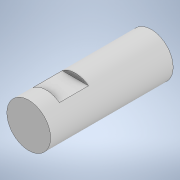
# Autodesk Inventor part: Eje_engrane
Saved by Autodesk Inventor 2021 (Build 250183000, 183)
## iProperties
Created: 2021-02-07
Part Number: Eje_engrane
Material: Genérico
Document SubType Name: Modeling
Designer: rotje
Density: 1 g/cm^3
Appearance: Valor por defecto
Author: rotje
Autodesk Inventor part; units mm, degrees
ref_plane "YZ Plane" through (0, 0, 0) normal (1, 0, 0) x (0, 1, 0)
ref_plane "XZ Plane" through (0, 0, 0) normal (0, 1, 0) x (-1, 0, 0)
sketch "Boceto1" plane through (0, 0, 0) normal (0, 0, 1) x (1, 0, 0)
  circle A0 centre (0, 0) radius 7.5
  dimension "d0" = 15
  constraints: 1 centre point, 1 coincident
  measures "d0" diameter of A0
extrude "Extrusión1" add sketch "Boceto1" along normal mid plane 42
ref_plane "Plano de trabajo1" through (0, 0, 5) normal (0, 0, 1) x (1, 0, 0)
sketch "Boceto3" plane through (0, 0, 5) normal (0, 0, 1) x (1, 0, 0)
  circle A0 centre (0, 0) radius 7.5 projected
  line L0 (0, 7.5) -> (0, 6)
  line L1 (0, 6) -> (4.5, 6)
  line L2 (0, 6) -> (-4.5, 6)
  dimension "d4" = 1.5
  constraints: 6 end point, 3 point on circle, 1 horizontal, 1 perpendicular, 1 vertical
  measures "d4" distance of L0.start L0.end
extrude "Extrusión2" cut sketch "Boceto3" along normal blind 10 contours L1 L0 A0 | A0 L0 L2
